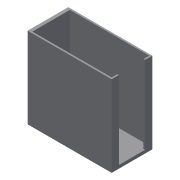
# Autodesk Inventor part: SteerServoInsert
Saved by Autodesk Inventor 2013 (Build 170138000, 138)
## iProperties
Created: 2012-05-21
Part Number: SteerServoInsert
Material: Generic
Document SubType Name: Modeling
Designer: dgitz
Density: 1 g/cm^3
Author: dgitz
Autodesk Inventor part; units mm, degrees
ref_plane "YZ Plane" through (0, 0, 0) normal (1, 0, 0) x (0, 1, 0)
ref_plane "XZ Plane" through (0, 0, 0) normal (0, 1, 0) x (-1, 0, 0)
ref_plane "XY Plane" through (0, 0, 0) normal (0, 0, 1) x (1, 0, 0)
sketch "Sketch2" plane through (0, 0, 0) normal (0, 0, 1) x (1, 0, 0)
  line L0 (-43.942, 43.18) -> (-43.942, 15.24)
  line L1 (-43.942, 15.24) -> (-36.322, 15.24)
  line L2 (-36.322, 15.24) -> (-25.4, 0)
  line L3 (-25.4, 0) -> (0, 0)
  line L4 (0, 0) -> (0, 43.18)
  line L5 (0.889, 43.18) -> (0.889, -1.778)
  line L6 (0.889, -1.778) -> (-45.72, -1.778)
  line L7 (-45.72, -1.778) -> (-45.72, 43.18)
  line L8 (-45.72, 43.18) -> (-43.942, 43.18)
  line L9 (0, 43.18) -> (0.889, 43.18)
  dimension "d1" = 7.62
  dimension "d2" = 27.94
  dimension "d3" = 10.922
  dimension "d4" = 43.18
  dimension "d5" = 1.778
  dimension "d6" = 0.889
  dimension "d7" = 1.778
  dimension "d10" = 44.958
  dimension "d11" = 46.609
  constraints: 20 end point, 4 parallel, 3 perpendicular, 1 coincident, 1 vertical
  measures "d1" distance of L0.end L1.end
  measures "d2" distance of L0.start L0.end
  measures "d3" horizontal distance of L1.end L2.end
  measures "d4" distance of L3.end L4.end
  measures "d5" distance between parallel lines of L7 L0
  measures "d6" distance between parallel lines of L5 L4
  measures "d7" distance between parallel lines of L6 L3
  measures "d10" distance from line of L0.start L6
  measures "d11" distance between parallel lines of L5 L7
extrude "Extrusion1" add sketch "Sketch2" along normal mid plane 20.828
sketch "Sketch5" plane through (0.889, -1.778, 10.414) normal (1, 0, 0) x (0, 0, -1)
  line L0 (0, 44.958) -> (20.828, 44.958) projected
  line L1 (3.175, 44.958) -> (17.653, 44.958)
  line L2 (17.653, 44.958) -> (17.653, 1.778)
  line L3 (17.653, 1.778) -> (3.175, 1.778)
  line L4 (3.175, 1.778) -> (3.175, 44.958)
  line L5 (0, 1.778) -> (20.828, 1.778) projected
  line L6 (0, 44.958) -> (20.828, 1.778) construction
  line L7 (3.175, 1.778) -> (17.653, 44.958) construction
  point P0 (10.414, 1.778)
  point P1 (10.414, 23.368)
  dimension "d14" = 14.478
  constraints: 12 end point, 2 midpoint, 2 parallel, 2 point on line, 1 horizontal, 1 perpendicular
  measures "d14" distance of L1.start L1.end
extrude "Extrusion2" cut sketch "Sketch5" against normal up to next
sketch "Sketch6" plane through (0, 0, 10.414) normal (0, 0, 1) x (1, 0, 0)
  line L0 (-45.72, 43.18) -> (0.889, 43.18)
  line L1 (0.889, 43.18) -> (0.889, -1.778)
  line L2 (0.889, -1.778) -> (-45.72, -1.778)
  line L3 (-45.72, -1.778) -> (-45.72, 43.18)
  constraints: 8 end point, 2 parallel, 1 horizontal, 1 perpendicular
extrude "Extrusion3" add sketch "Sketch6" along normal blind 0.889
mirror "Mirror1" about plane through (0, 0, 0) normal (0, 0, 1) of "Extrusion3"
body "Solid1"
